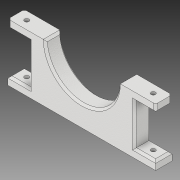
# Autodesk Inventor part: 2121_Copper Tube Clamp Bottom_V1
Saved by Autodesk Inventor 2020 (Build 240168000, 168)
## iProperties
Created: 2017-06-29
Part Number: 2121_Copper Tube Clamp Bottom_V1
Material: ABS Plastic
Document SubType Name: Modeling
Designer: MPI
Density: 1.06 g/cm^3
Appearance: Smooth - White
Mass: 298.455 g
Surface Area: 441.503 cm^2
Volume: 281.562 cm^3
Author: MPI
Autodesk Inventor part; units mm, degrees
ref_plane "YZ Plane" through (0, 0, 0) normal (1, 0, 0) x (0, 1, 0)
ref_plane "XZ Plane" through (0, 0, 0) normal (0, 1, 0) x (-1, 0, 0)
ref_plane "XY Plane" through (0, 0, 0) normal (0, 0, 1) x (1, 0, 0)
sketch "Sketch1" plane through (0, 0, 0) normal (0, 0, 1) x (1, 0, 0)
  arc A0 (-56.515, 0) -> (56.515, 0) centre (0, 0) ccw
  line L0 (114.3, -88.9) -> (-114.3, -88.9)
  line L1 (-114.3, 88.9) -> (114.3, 88.9) construction
  line L2 (-56.515, 0) -> (-114.3, 0)
  line L3 (-114.3, -76.2) -> (-81.5672, -76.2)
  line L4 (81.5672, -76.2) -> (114.3, -76.2)
  line L5 (114.3, 0) -> (114.3, -12.7)
  line L6 (114.3, -76.2) -> (114.3, -88.9)
  line L7 (-114.3, -88.9) -> (-114.3, -76.2)
  line L8 (-114.3, -12.7) -> (-114.3, 0)
  line L9 (-114.3, 0) -> (-56.515, 0)
  line L10 (56.515, 0) -> (114.3, 0)
  line L11 (-114.3, -12.7) -> (-81.5672, -12.7)
  line L12 (81.5672, -12.7) -> (114.3, -12.7)
  line L13 (-81.5672, -12.7) -> (-81.5672, -76.2)
  line L14 (81.5672, -12.7) -> (81.5672, -76.2)
  dimension "d0" = 113.03
  dimension "d7" = 57.785
  constraints: 30 end point, 10 perpendicular, 6 equal length, 3 horizontal, 2 coincident, 2 point on circle, 1 centre point
  measures "d0" diameter of A0
  measures "d7" distance of L2.start L2.end
extrude "Extrusion1" add sketch "Sketch1" along normal blind 25.4
sketch "Sketch2" plane through (81.5672, -12.7, 0) normal (0, -1, 0) x (1, 0, 0)
  line L0 (32.7328, 0) -> (0, 25.4) construction
  line L1 (-195.8672, 0) -> (-195.8672, 25.4) projected
  line L2 (-195.8672, 25.4) -> (-163.1345, 0) construction
  point P0 (-81.5672, 0)
  point P1 (-179.5008, 12.7)
  point P2 (16.3664, 12.7)
  constraints: 4 end point, 2 midpoint
hole "Hole1" at (-97.9336, -12.7, 12.7) at (97.9336, -12.7, 12.7) direction (0, -1, 0) diameter 6.604 end through all clearance for "Flat Head Machine Screw" size "M6" standard "Ansi Metric M Profile"
sketch "Sketch3" plane through (-114.3, -88.9, 0) normal (0, -1, 0) x (1, 0, 0)
  circle A0 centre (212.2336, 12.7) radius 3.302 projected
  circle A1 centre (16.3664, 12.7) radius 3.302 projected
  point P0 (114.3, 0)
  constraints: 2 coincident
hole "Hole2" at (97.9336, -88.9, 12.7) at (-97.9336, -88.9, 12.7) direction (0, 1, 0) diameter 6.7564 end through all clearance for "Flat Head Machine Screw (82)" size "1/4" standard "Ansi Unified Screw Threads"
sketch "Sketch4" plane through (-114.3, -12.7, 0) normal (0, -1, 0) x (1, 0, 0)
  circle A0 centre (16.3664, 12.7) radius 3.3782 projected
  circle A1 centre (16.3664, 12.7) radius 4.318
  circle A2 centre (212.2336, 12.7) radius 3.3782 projected
  circle A3 centre (212.2336, 12.7) radius 4.318
  point P0 (114.3, 0)
  dimension "d26" = 8.636
  dimension "d27" = 8.636
  constraints: 2 centre point, 2 coincident
  measures "d26" diameter of A1
  measures "d27" diameter of A3
extrude "Extrusion2" cut sketch "Sketch4" against normal blind 8.382
chamfer "Chamfer1" distance 3.175 angle 45 6 edges at (-56.515, 0, 12.7) (56.515, 0, 12.7) (-114.3, -6.35, 25.4) (-114.3, -6.35, 0) (114.3, -6.35, 25.4) (114.3, -6.35, 0)
chamfer "Chamfer2" distance 3.175 angle 45 18 edges at (0, -56.515, 25.4) (0, -56.515, 0) (-81.5672, -44.45, 25.4) (-96.3461, -12.7, 25.4) (-81.5672, -44.45, 0) (-96.3461, -12.7, 0) (-114.3, -12.7, 12.7) (-97.9336, -76.2, 25.4) (-97.9336, -76.2, 0) (-114.3, -76.2, 12.7) (81.5672, -44.45, 25.4) (81.5672, -44.45, 0) (96.3461, -12.7, 25.4) (114.3, -12.7, 12.7) (96.3461, -12.7, 0) (97.9336, -76.2, 25.4) (114.3, -76.2, 12.7) (97.9336, -76.2, 0)
body "Solid1"
